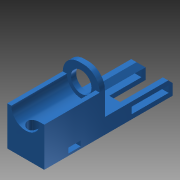
# Autodesk Inventor part: Solinoid holder v5
Saved by Autodesk Inventor 2013 SP2 (Build 170200200, 200)
## iProperties
Created: 2017-05-28
Part Number: Solinoid holder v5
Material: Generic
Document SubType Name: Modeling
Designer: hdv
Density: 1 g/cm^3
Author: hdv
Autodesk Inventor part; units mm, degrees
ref_plane "YZ Plane" through (0, 0, 0) normal (1, 0, 0) x (0, 1, 0)
ref_plane "XZ Plane" through (0, 0, 0) normal (0, 1, 0) x (-1, 0, 0)
ref_plane "XY Plane" through (0, 0, 0) normal (0, 0, 1) x (1, 0, 0)
sketch "Sketch1" plane through (0, 0, 0) normal (0, 0, 1) x (1, 0, 0)
  circle A0 centre (0, 0) radius 7
  circle A1 centre (0, 0) radius 5
  circle A2 centre (0, 0) radius 1
  line L0 (-9, 0) -> (9, 0)
  line L1 (9, 0) -> (9, -19)
  line L2 (9, -19) -> (-9, -19)
  line L3 (-9, -19) -> (-9, 0)
  dimension "d11" = 14
  dimension "d12" = 10
  dimension "d13" = 2
  dimension "d18" = 19
  dimension "d19" = 18
  constraints: 8 end point, 5 coincident, 3 centre point, 2 parallel, 1 horizontal, 1 midpoint, 1 perpendicular
  measures "d11" diameter of A0
  measures "d12" diameter of A1
  measures "d13" diameter of A2
  measures "d18" distance of L2.end L0.start
  measures "d19" distance of L1.end L2.end
extrude "Extrusion1" add sketch "Sketch1" along normal blind 27 contours L0 L1 L2 L3 A0 | A0 L0 A1 | A1 L0 A2 | A2 L0 picked at (6.2655, -0.5584) picked at (3.6182, -0.3989) picked at (-0.2952, -0.1549)
sketch "Sketch3" plane through (0, 0, 0) normal (0, 0, -1) x (-1, 0, 0)
  line L0 (9, -19) -> (9, 0) projected
  line L1 (-9, -19) -> (9, -19)
  line L2 (9, -19) -> (9, 8)
  line L3 (9, 8) -> (-9, 8)
  line L4 (-9, 8) -> (-9, -19)
  dimension "d22" = 27
  constraints: 8 end point, 2 parallel, 1 collinear, 1 horizontal, 1 perpendicular
  measures "d22" distance of L1.end L2.end
extrude "Extrusion6" add sketch "Sketch3" along normal blind 2.5
extrude "Extrusion5" cut sketch "Sketch1" along normal blind 30 contours L0 A1 A0 | A0 L0 A1 | L0 A2 A1 | A1 L0 A2 | L0 A2 | A2 L0
extrude "Extrusion7" cut sketch "Sketch1" against normal through all contours L0 A2 A1 | A1 L0 A2 | L0 A2 | A2 L0
fillet "Fillet1" radius 8 2 edges at (-9, 8, -1.25) (9, 8, -1.25)
sketch "Sketch4" plane through (9, -19, 27) normal (1, 0, 0) x (0, 0, -1)
  line L0 (0, 0) -> (29.5, 0) projected
  line L1 (11.75, 3.5) -> (17.75, 3.5)
  line L2 (17.75, 3.5) -> (17.75, 1)
  line L3 (17.75, 1) -> (11.75, 1)
  line L4 (11.75, 1) -> (11.75, 3.5)
  point P0 (14.75, 0)
  point P1 (14.75, 1)
  dimension "d32" = 6
  dimension "d33" = 2.5
  dimension "d34" = 1
  constraints: 8 end point, 2 midpoint, 2 parallel, 1 horizontal, 1 perpendicular, 1 vertical alignment
  measures "d32" distance of L2.end L3.end
  measures "d33" distance of L1.end L2.end
  measures "d34" distance between parallel lines of L0 L3
extrude "Extrusion8" cut sketch "Sketch4" against normal through all
sketch "Sketch5" plane through (0, 0, -2.5) normal (0, 0, -1) x (-1, 0, 0)
  line L0 (9, -19) -> (9, 0) projected
  line L1 (-9, -19) -> (9, -19)
  line L2 (9, -19) -> (9, -11.5)
  line L3 (9, -11.5) -> (-9, -11.5)
  line L4 (-9, -11.5) -> (-9, -19)
  dimension "d37" = 7.5
  constraints: 8 end point, 2 parallel, 1 horizontal, 1 perpendicular, 1 point on line
  measures "d37" distance of L2.end L1.end
extrude "Extrusion9" add sketch "Sketch5" along normal blind 33
sketch "Sketch6" plane through (-9, -11.5, -2.5) normal (0, 1, 0) x (1, 0, 0)
  line L0 (4.8, 10) -> (13.2, 10)
  line L1 (13.2, 10) -> (13.2, 33)
  line L2 (13.2, 33) -> (4.8, 33)
  line L3 (4.8, 33) -> (4.8, 10)
  line L4 (0, 33) -> (18, 33) projected
  point P0 (9, -2.5)
  point P1 (9, 33)
  point P2 (9, 33)
  dimension "d45" = 23
  dimension "d47" = 0
  dimension "d69" = 8.4
  constraints: 8 end point, 2 midpoint, 2 parallel, 1 coincident, 1 horizontal, 1 perpendicular
  measures "d45" distance of L2.end L0.start
  measures "d47" distance between parallel lines of L4 L2
  measures "d69" distance of L0.start L0.end
extrude "Extrusion10" cut sketch "Sketch6" against normal blind 30
sketch "Sketch7" plane through (9, -19, 27) normal (1, 0, 0) x (0, 0, -1)
  line L0 (42.5, 5.35) -> (60.5, 5.35)
  line L1 (60.5, 5.35) -> (60.5, 2.15)
  line L2 (60.5, 2.15) -> (42.5, 2.15)
  line L3 (42.5, 2.15) -> (42.5, 5.35)
  line L4 (62.5, 7.5) -> (62.5, 0) projected
  line L5 (62.5, 7.5) -> (39.5, 7.5) projected
  point P0 (27, 19)
  point P1 (60.5, 3.75)
  point P2 (62.5, 3.75)
  point P3 (51.5, 5.35)
  point P4 (51, 7.5)
  point P5 (59.5, 7.5)
  dimension "d49" = 3.2
  dimension "d55" = 18
  dimension "d70" = 20
  constraints: 8 end point, 4 midpoint, 2 parallel, 1 horizontal, 1 horizontal alignment, 1 perpendicular
  measures "d49" distance of L2.end L0.start
  measures "d55" distance of L0.start L0.end
  measures "d70" distance between parallel lines of L4 L3
extrude "Extrusion11" cut sketch "Sketch7" against normal through all
sketch "Sketch8" plane through (-9, -11.5, -2.5) normal (0, 1, 0) x (1, 0, 0)
  circle A0 centre (9, 4.5) radius 3
  circle A1 centre (9, -25.5) radius 3
  line L0 (16, -29.5) -> (2, -29.5) projected
  point P0 (9, -2.5)
  dimension "d56" = 6
  dimension "d57" = 6
  dimension "d58" = 4
  dimension "d59" = 34
  constraints: 2 centre point, 1 vertical alignment
  measures "d56" diameter of A0
  measures "d57" diameter of A1
  measures "d58" distance from line of A1.centre L0
  measures "d59" distance from line of L0 A0.centre
extrude "Extrusion12" cut sketch "Sketch8" along normal mid plane 11
sketch "Sketch9" plane through (0, -17, -7) normal (0, 1, 0) x (1, 0, 0)
  circle A0 centre (0, 0) radius 3 projected
  circle A1 centre (0, 0) radius 1.6
  circle A2 centre (0, -30) radius 1.6
  point P0 (0, -7)
  dimension "d62" = 3.2
  dimension "d63" = 3.2
  constraints: 2 centre point, 1 coincident, 1 other
  measures "d62" diameter of A1
  measures "d63" diameter of A2
extrude "Extrusion13" cut sketch "Sketch9" against normal through all contours A1 | A2
chamfer "Chamfer2" distance 2.2 angle 45 4 edges at (4.2, -11.5, -24) (-4.2, -11.5, -24) (6.6, -11.5, -35.5) (-6.6, -11.5, -35.5)
body "Solid1"
